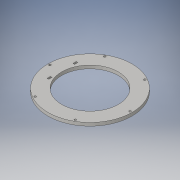
# Autodesk Inventor part: Turntable Outer Gear
Saved by Autodesk Inventor 2016 (Build 200138000, 138)
## iProperties
Created: 2016-04-25
Part Number: Turntable Outer Gear
Material: Generic
Document SubType Name: Modeling
Designer: rubenjm
Density: 1 g/cm^3
Appearance: Default
Author: rubenjm
Autodesk Inventor part; units mm, degrees
ref_plane "YZ Plane" through (0, 0, 0) normal (1, 0, 0) x (0, 1, 0)
ref_plane "XZ Plane" through (0, 0, 0) normal (0, 1, 0) x (-1, 0, 0)
ref_plane "XY Plane" through (0, 0, 0) normal (0, 0, 1) x (1, 0, 0)
sketch "Sketch1" plane through (0, 0, 0) normal (0, 1, 0) x (-1, 0, 0)
  circle A0 centre (0, 0) radius 165.1
  circle A1 centre (0, 0) radius 111.125
  line L0 (-117.475, 63.5) -> (-111.125, 63.5) construction
  line L1 (-111.125, 63.5) -> (-111.125, 50.8) construction
  line L2 (-111.125, 50.8) -> (-117.475, 50.8) construction
  line L3 (-117.475, 50.8) -> (-117.475, 63.5) construction
  line L4 (-111.125, 50.8) -> (-111.125, -50.8) construction
  line L5 (-111.125, 50.8) -> (-212.725, 50.8) construction
  line L6 (-111.125, -50.8) -> (-117.475, -50.8) construction
  line L7 (-117.475, -50.8) -> (-117.475, -38.1) construction
  line L8 (-117.475, -38.1) -> (-111.125, -38.1) construction
  line L9 (-111.125, -38.1) -> (-111.125, -50.8) construction
  line L10 (-111.125, 0) -> (-60.325, 0) construction
  line L11 (-111.125, 0) -> (-60.325, 0) construction
  circle A2 centre (0, 0) radius 60.325 construction
  line L12 (0, 0) -> (-60.325, 0) construction
  dimension "d0" = 330.2
  dimension "d1" = 222.25
  dimension "d21" = 6.35
  dimension "d22" = 12.7
  dimension "d23" = 101.6
  dimension "d24" = 90
  dimension "d25" = 6.35
  dimension "d26" = 12.7
  dimension "d27" = 50.8
  dimension "d28" = 0
  constraints: 26 end point, 4 parallel, 3 coincident, 3 horizontal, 2 centre point, 2 equal length, 2 perpendicular, 1 horizontal alignment, 1 midpoint, 2 other
  measures "d0" diameter of A0
  measures "d1" diameter of A1
  measures "d21" distance of L2.start L2.end
  measures "d22" distance of L0.end L2.start
  measures "d23" distance of L2.start L6.start
  measures "d24" angle of L5 L4
  measures "d25" distance of L8.start L8.end
  measures "d26" distance of L6.end L8.start
  measures "d27" distance of L10.start L10.end
  measures "d28" distance between parallel lines of L10 L11
extrude "Extrusion1" add sketch "Sketch1" along normal blind 12.7
sketch "Sketch2" plane through (0, 12.7, 0) normal (0, 1, 0) x (1, 0, 0)
  line L0 (-117.475, 63.5) -> (-111.125, 63.5)
  line L1 (-111.125, 63.5) -> (-111.125, 50.8)
  line L2 (-111.125, 50.8) -> (-117.475, 50.8)
  line L3 (-117.475, 50.8) -> (-117.475, 63.5)
  line L4 (-111.125, 50.8) -> (-111.125, -50.8) construction
  line L5 (-111.125, 50.8) -> (-212.725, 50.8) construction
  line L6 (-111.125, -50.8) -> (-117.475, -50.8)
  line L7 (-117.475, -50.8) -> (-117.475, -38.1)
  line L8 (-117.475, -38.1) -> (-111.125, -38.1)
  line L9 (-111.125, -38.1) -> (-111.125, -50.8)
  line L10 (-111.125, 0) -> (-60.325, 0) construction
  line L11 (-111.125, 0) -> (-60.325, 0) construction
  circle A0 centre (0, 0) radius 60.325 construction
  line L12 (0, 0) -> (-60.325, 0) construction
  dimension "d4" = 6.35
  dimension "d5" = 12.7
  dimension "d6" = 101.6
  dimension "d7" = 90
  dimension "d8" = 6.35
  dimension "d9" = 12.7
  dimension "d10" = 50.8
  dimension "d11" = 0
  constraints: 26 end point, 4 parallel, 3 horizontal, 2 equal length, 2 perpendicular, 1 coincident, 1 horizontal alignment, 1 midpoint, 2 other
  measures "d4" distance of L1.end L2.end
  measures "d5" distance of L0.end L1.end
  measures "d6" distance of L1.end L4.end
  measures "d7" angle of L5 L4
  measures "d8" distance of L7.end L8.end
  measures "d9" distance of L6.end L7.end
  measures "d10" distance of L10.start L10.end
  measures "d11" distance between parallel lines of L10 L11
extrude "Extrusion2" cut sketch "Sketch2" against normal through all
sketch "Sketch3" plane through (0, 12.7, 0) normal (0, 1, 0) x (1, 0, 0)
  circle A0 centre (0, 0) radius 157.48 construction
  circle A1 centre (-157.48, 0) radius 3.9687
  circle A2 centre (-78.74, -136.3817) radius 3.9687
  circle A3 centre (78.74, -136.3817) radius 3.9687
  circle A4 centre (157.48, 0) radius 3.9687
  circle A5 centre (78.74, 136.3817) radius 3.9687
  circle A6 centre (-78.74, 136.3817) radius 3.9687
  dimension "d16" = 314.96
  dimension "d17" = 7.9375
  dimension "d18" = 360
  constraints: 6 centre point, 1 coincident, 1 horizontal alignment, 15 other
  measures "d17" diameter of A1
extrude "Extrusion3" cut sketch "Sketch3" against normal through all
equation "\"d21\" = d25"
equation "\"d4\" = d8"
body "Solid1"
